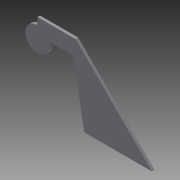
# Autodesk Inventor part: Arm
Saved by Autodesk Inventor 2014 (Build 180170000, 170)
## iProperties
Created: 2016-09-28
Part Number: Arm
Material: Generic
Document SubType Name: Modeling
Designer: choices
Density: 1 g/cm^3
Appearance: Default
Author: choices
Autodesk Inventor part; units mm, degrees
ref_plane "YZ Plane" through (0, 0, 0) normal (1, 0, 0) x (0, 1, 0)
ref_plane "XZ Plane" through (0, 0, 0) normal (0, 1, 0) x (-1, 0, 0)
ref_plane "XY Plane" through (0, 0, 0) normal (0, 0, 1) x (1, 0, 0)
sketch "Sketch1" plane through (0, 0, 0) normal (0, 0, 1) x (1, 0, 0)
  circle A0 centre (0, 0) radius 44.45
  line L0 (0, 44.45) -> (0, 69.85)
  line L1 (0, 69.85) -> (139.7, 69.85)
  line L2 (139.7, 69.85) -> (419.1, -209.55)
  line L3 (419.1, -209.55) -> (170.6858, -209.55)
  line L4 (131.4971, 12.7) -> (42.5971, 12.7)
  line L5 (131.4971, 12.7) -> (170.6858, -209.55)
  dimension "d0" = 88.9
  dimension "d1" = 25.4
  dimension "d2" = 139.7
  dimension "d3" = 88.9
  dimension "d4" = 135
  dimension "d6" = 279.4
  dimension "d7" = 0
  dimension "d8" = 12.7
  dimension "d9" = 100
  constraints: 12 end point, 2 parallel, 2 point on circle, 1 centre point, 1 coincident, 1 perpendicular, 1 vertical
  measures "d0" diameter of A0
  measures "d1" distance of L0.start L0.end
  measures "d2" distance of L0.end L1.end
  measures "d3" distance of L4.start L4.end
  measures "d4" angle of L2 L1
  measures "d6" distance between parallel lines of L3 L1
  measures "d7" distance from line of point (0, 0) L0
  measures "d8" distance from line of point (0, 0) L4
  measures "d9" angle of L5 L4
extrude "Extrusion1" add sketch "Sketch1" along normal blind 9.525
body "Solid1"
